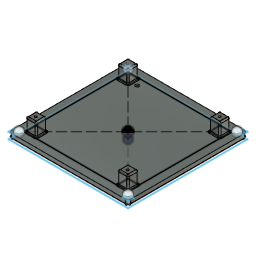
BuzzerBot (Autodesk Fusion 360 design; units mm, degrees)
Autodesk Fusion 360 part; units mm, degrees
note: some values were not read from the file. Set by a fixed rule: which sketch regions a step uses.
sketch "Sketch15" plane through (0, 0, 0) normal (0, 0, 1) x (1, 0, 0)
  line L0 (45.45, 45.45) -> (-45.45, 45.45)
  line L1 (-45.45, 45.45) -> (-45.45, -45.45)
  line L2 (-45.45, -45.45) -> (45.45, -45.45)
  line L3 (45.45, -45.45) -> (45.45, 45.45)
  dimension "d68" = 90.9
  dimension "d69" = 90.9
  constraint horizontal L0
  constraint perpendicular L0 L1
  constraint parallel L0 L2
  constraint parallel L1 L3
  measures "d68" distance of L1.end L2.end
  measures "d69" distance of L0.end L1.end
extrude "Extrude9" add sketch "Sketch15" along normal blind 5
sketch "Sketch16" plane through (0, 0, 5) normal (0, 0, 1) x (-1, 0, 0)
  line L0 (-45.45, 45.45) -> (-45.45, -45.45)
  line L1 (-45.45, -45.45) -> (45.45, -45.45)
  line L2 (45.45, -45.45) -> (45.45, 45.45)
  line L3 (45.45, 45.45) -> (-45.45, 45.45)
  line L4 (-39.45, -39.45) -> (39.45, -39.45)
  line L5 (39.45, -39.45) -> (39.45, 39.45)
  line L6 (39.45, 39.45) -> (-39.45, 39.45)
  line L7 (-39.45, 39.45) -> (-39.45, -39.45)
  line L8 (-39.45, -39.45) -> (39.45, 39.45) construction
  line L9 (39.45, -39.45) -> (-39.45, 39.45) construction
  line L10 (39.45, -39.45) -> (30.95, -39.45)
  line L11 (30.95, -39.45) -> (30.95, -30.95)
  line L12 (30.95, -30.95) -> (39.45, -30.95)
  line L13 (39.45, -30.95) -> (39.45, -39.45)
  line L14 (-39.45, -39.45) -> (-30.95, -39.45)
  line L15 (-30.95, -39.45) -> (-30.95, -30.95)
  line L16 (-30.95, -30.95) -> (-39.45, -30.95)
  line L17 (-39.45, -30.95) -> (-39.45, -39.45)
  line L18 (39.45, 39.45) -> (30.95, 39.45)
  line L19 (30.95, 39.45) -> (30.95, 30.95)
  line L20 (30.95, 30.95) -> (39.45, 30.95)
  line L21 (39.45, 30.95) -> (39.45, 39.45)
  line L22 (-39.45, 39.45) -> (-30.95, 39.45)
  line L23 (-30.95, 39.45) -> (-30.95, 30.95)
  line L24 (-30.95, 30.95) -> (-39.45, 30.95)
  line L25 (-39.45, 30.95) -> (-39.45, 39.45)
  line L26 (30.95, -30.95) -> (38.95, -30.95)
  line L27 (38.95, -30.95) -> (38.95, -38.95)
  line L28 (38.95, -38.95) -> (30.95, -38.95)
  line L29 (30.95, -38.95) -> (30.95, -30.95)
  line L30 (-30.95, -30.95) -> (-38.95, -30.95)
  line L31 (-38.95, -30.95) -> (-38.95, -38.95)
  line L32 (-38.95, -38.95) -> (-30.95, -38.95)
  line L33 (-30.95, -38.95) -> (-30.95, -30.95)
  line L34 (30.95, 30.95) -> (38.95, 30.95)
  line L35 (38.95, 30.95) -> (38.95, 38.95)
  line L36 (38.95, 38.95) -> (30.95, 38.95)
  line L37 (30.95, 38.95) -> (30.95, 30.95)
  line L38 (-30.95, 30.95) -> (-38.95, 30.95)
  line L39 (-38.95, 30.95) -> (-38.95, 38.95)
  line L40 (-38.95, 38.95) -> (-30.95, 38.95)
  line L41 (-30.95, 38.95) -> (-30.95, 30.95)
  dimension "d72" = 78.9
  dimension "d73" = 78.9
  dimension "d74" = 8.5
  dimension "d75" = 8.5
  dimension "d76" = 8.5
  dimension "d77" = 8.5
  dimension "d78" = 8.5
  dimension "d79" = 8.5
  dimension "d80" = 8.5
  dimension "d81" = 8.5
  dimension "d82" = 8
  dimension "d83" = 8
  dimension "d84" = 8
  dimension "d85" = 8
  dimension "d86" = 8
  dimension "d87" = 8
  dimension "d88" = 8
  dimension "d89" = 8
  constraint horizontal L4
  constraint perpendicular L4 L5
  constraint parallel L4 L6
  constraint parallel L5 L7
  constraint coincident L8 origin
  constraint coincident L9 origin
  constraint horizontal L10
  constraint vertical L11
  constraint horizontal L12
  constraint vertical L13
  constraint horizontal L14
  constraint vertical L15
  constraint horizontal L16
  constraint vertical L17
  constraint horizontal L18
  constraint vertical L19
  constraint horizontal L20
  constraint vertical L21
  constraint horizontal L22
  constraint vertical L23
  constraint horizontal L24
  constraint vertical L25
  constraint horizontal L26
  constraint vertical L27
  constraint horizontal L28
  constraint vertical L29
  constraint horizontal L30
  constraint vertical L31
  constraint horizontal L32
  constraint vertical L33
  constraint horizontal L34
  constraint vertical L35
  constraint horizontal L36
  constraint vertical L37
  constraint horizontal L38
  constraint vertical L39
  constraint horizontal L40
  constraint vertical L41
  measures "d72" distance of L5.end L6.end
  measures "d73" distance of L4.end L5.end
  measures "d74" distance of L4.end L10.end
  measures "d75" distance of L4.end L12.end
  measures "d76" distance of L4.start L14.end
  measures "d77" distance of L4.start L16.end
  measures "d78" distance of L5.end L18.end
  measures "d79" distance of L5.end L20.end
  measures "d80" distance of L6.end L22.end
  measures "d81" distance of L6.end L24.end
  measures "d82" distance of L11.end L26.end
  measures "d83" distance of L11.end L28.end
  measures "d84" distance of L15.end L30.end
  measures "d85" distance of L15.end L32.end
  measures "d86" distance of L19.end L34.end
  measures "d87" distance of L19.end L36.end
  measures "d88" distance of L23.end L38.end
  measures "d89" distance of L23.end L40.end
extrude "Extrude10" add sketch "Sketch16" along normal blind 10 contours L15 L16 L30 L31 L32 L33 | L11 L12 L26 L27 L28 L29 | L23 L24 L38 L39 L40 L41 | L19 L20 L34 L35 L36 L37
sketch "Sketch17" plane through (0, 0, 15) normal (0, 0, 1) x (-1, 0, 0)
  line L0 (39.4192, -39.4543) -> (35.3192, -39.4543)
  line L1 (39.4192, -36.5543) -> (39.4192, -39.4543)
  circle A0 centre (35.0497, -34.7418) radius 0.85
  circle A1 centre (-34.95, -34.95) radius 0.85
  line L2 (34.1997, -34.7461) -> (-34.1, -34.9542)
  line L3 (-30.95, -38.95) -> (-30.95, -30.95)
  line L4 (-30.95, -30.95) -> (-38.95, -30.95)
  line L5 (-38.95, -30.95) -> (-38.95, -38.95)
  line L6 (-38.95, -38.95) -> (-30.95, -38.95)
  line L7 (39.0497, -38.7418) -> (35.0497, -38.7418)
  line L8 (39.0497, -34.7418) -> (39.0497, -38.7418)
  line L9 (-38.95, -38.95) -> (-34.95, -38.95)
  line L10 (-34.95, -38.95) -> (-34.95, -34.95)
  line L11 (-34.95, -34.95) -> (-38.95, -34.95)
  line L12 (-38.95, -34.95) -> (-38.95, -38.95)
  circle A2 centre (35.0497, 35.2582) radius 0.85
  circle A3 centre (-34.9503, 35.2582) radius 0.85
  line L13 (35.0497, -33.8918) -> (35.0497, 34.4082)
  line L14 (34.1997, 35.2582) -> (-34.1003, 35.2582)
  dimension "d92" = 4.1
  dimension "d93" = 2.9
  dimension "d94" = 1.7
  dimension "d95" = 70
  dimension "d97" = 1.7
  dimension "d130" = 4
  dimension "d131" = 4
  dimension "d134" = 4
  dimension "d135" = 4
  dimension "d136" = 70
  dimension "d137" = 1.7
  dimension "d138" = 70
  dimension "d139" = 1.7
  constraint horizontal L0
  constraint vertical L1
  constraint coincident A0 L2.start
  constraint coincident A1 L2.end
  constraint horizontal L7
  constraint vertical L8
  constraint horizontal L9
  constraint vertical L10
  constraint horizontal L11
  constraint vertical L12
  constraint coincident L5.end L6.start
  constraint coincident A1.centre L10.end
  constraint coincident A0 L13.start
  constraint coincident A2 L13.end
  constraint coincident A2 L14.start
  constraint coincident A3 L14.end
  measures "d92" distance of L0.start L0.end
  measures "d93" distance of L0.start L1.start
  measures "d94" diameter of A0
  measures "d95" distance of A0.centre A1.centre
  measures "d97" diameter of A1
  measures "d130" distance of L7.start L7.end
  measures "d131" distance of L7.start L8.start
  measures "d134" distance of L5.end L9.end
  measures "d135" distance of L5.end L11.end
  measures "d136" distance of A0.centre A2.centre
  measures "d137" diameter of A2
  measures "d138" distance of A2.centre A3.centre
  measures "d139" diameter of A3
extrude "Extrude11" cut sketch "Sketch17" against normal blind 11 contours A0 | A1 L10 L11 | A1 L10 L11
sketch "Sketch18" plane through (0, 0, 5) normal (0, 0, 1) x (-1, 0, 0)
  line L0 (-45.5, -45.5) -> (-41.5, -45.5)
  line L1 (-41.5, -45.5) -> (-41.5, -43.3)
  line L2 (-43.3, -41.5) -> (-45.5, -41.5)
  line L3 (-45.5, -41.5) -> (-45.5, -45.5)
  circle A0 centre (-41.5, -41.5) radius 1.8
  line L4 (45.5, -45.5) -> (41.5, -45.5)
  line L5 (41.5, -45.5) -> (41.5, -43.3)
  line L6 (43.3, -41.5) -> (45.5, -41.5)
  line L7 (45.5, -41.5) -> (45.5, -45.5)
  circle A1 centre (41.5, -41.5) radius 1.8
  line L8 (45.5, 45.5) -> (41.5, 45.5)
  line L9 (41.5, 45.5) -> (41.5, 43.3)
  line L10 (43.3, 41.5) -> (45.5, 41.5)
  line L11 (45.5, 41.5) -> (45.5, 45.5)
  circle A2 centre (41.5, 41.5) radius 1.8
  line L12 (-45.5, 45.5) -> (-41.5, 45.5)
  line L13 (-45.5, 41.5) -> (-45.5, 45.5)
  circle A3 centre (-41.5, 41.5) radius 1.8
  line L14 (-41.5, 45.5) -> (-41.5, 43.3)
  line L15 (-43.3, 41.5) -> (-45.5, 41.5)
  dimension "d104" = 4
  dimension "d105" = 4
  dimension "d106" = 3.6
  dimension "d107" = 4
  dimension "d108" = 4
  dimension "d109" = 3.6
  dimension "d110" = 4
  dimension "d111" = 4
  dimension "d112" = 3.6
  dimension "d113" = 4
  dimension "d114" = 4
  dimension "d115" = 3.6
  constraint horizontal L0
  constraint vertical L1
  constraint horizontal L2
  constraint vertical L3
  constraint coincident A0 L2.start
  constraint coincident A0 L1.end
  constraint horizontal L4
  constraint vertical L5
  constraint horizontal L6
  constraint vertical L7
  constraint coincident A1 L6.start
  constraint coincident A1 L5.end
  constraint horizontal L8
  constraint vertical L9
  constraint horizontal L10
  constraint vertical L11
  constraint coincident A2 L9.end
  constraint coincident A2 L10.start
  constraint horizontal L12
  constraint vertical L13
  constraint coincident A3 L14.end
  constraint vertical L14
  constraint coincident A3 L15.start
  constraint horizontal L15
  measures "d104" distance of L0.start L0.end
  measures "d105" distance of L0.start L2.end
  measures "d106" diameter of A0
  measures "d107" distance of L4.start L4.end
  measures "d108" distance of L4.start L6.end
  measures "d109" diameter of A1
  measures "d110" distance of L8.start L8.end
  measures "d111" distance of L8.start L10.end
  measures "d112" diameter of A2
  measures "d113" distance of L12.start L12.end
  measures "d114" distance of L12.start L13.start
  measures "d115" diameter of A3
extrude "Extrude12" cut sketch "Sketch18" against normal blind 5 contours A0 | A1 | A2 | A3
fillet "Fillet4" radius 1 12 edges at (30.95, 34.95, 15) (34.95, 30.95, 15) (38.95, 34.95, 15) (34.95, 38.95, 15) (34.95, 38.95, 5) (30.95, 34.95, 5) (38.95, 38.95, 10) (30.95, 38.95, 10) (30.95, 30.95, 10) (34.95, 30.95, 5) (38.95, 30.95, 10) (38.95, 34.95, 5)
fillet "Fillet5" radius 1 12 edges at (-30.95, 34.95, 15) (-34.95, 30.95, 15) (-38.95, 34.95, 15) (-34.95, 38.95, 15) (-30.95, 38.95, 10) (-30.95, 30.95, 10) (-30.95, 34.95, 5) (-34.95, 30.95, 5) (-38.95, 30.95, 10) (-38.95, 38.95, 10) (-34.95, 38.95, 5) (-38.95, 34.95, 5)
fillet "Fillet6" radius 1 12 edges at (38.95, -38.95, 10) (34.95, -38.95, 5) (38.95, -34.95, 5) (38.95, -30.95, 10) (38.95, -34.95, 15) (34.95, -38.95, 15) (30.95, -38.95, 10) (30.95, -34.95, 15) (34.95, -30.95, 15) (30.95, -30.95, 10) (34.95, -30.95, 5) (30.95, -34.95, 5)
fillet "Fillet7" radius 1 12 edges at (-38.95, -30.95, 10) (-38.95, -34.95, 15) (-34.95, -30.95, 15) (-30.95, -30.95, 10) (-34.95, -30.95, 5) (-38.95, -34.95, 5) (-38.95, -38.95, 10) (-34.95, -38.95, 15) (-30.95, -34.95, 15) (-30.95, -38.95, 10) (-34.95, -38.95, 5) (-30.95, -34.95, 5)
fillet "Fillet8" radius 2 4 edges at (0, -45.45, 0) (45.45, 0, 0) (0, 45.45, 0) (-45.45, 0, 0)
fillet "Fillet9" radius 2 8 edges at (44.8642, -44.8642, 0.5858) (45.45, -45.45, 3.5) (-44.8642, -44.8642, 0.5858) (-45.45, -45.45, 3.5) (44.8642, 44.8642, 0.5858) (45.45, 45.45, 3.5) (-44.8642, 44.8642, 0.5858) (-45.45, 45.45, 3.5)
extrude "Extrude13" cut sketch "Sketch17" against normal blind 11 contours A2 | A3
cylinder "CylinderPrimitive1" cut diameter 2.828 height -1 placed x (1, 0, 0) y (0, 1, 0) z (0, 0, 1) at (-27, 34, 5)
